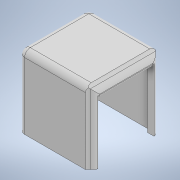
# Autodesk Inventor part: NEMA17_Shroud
Saved by Autodesk Inventor 2021 (Build 250183000, 183)
## iProperties
Created: 2021-10-06
Part Number: NEMA17_Shroud
Material: Generic
Document SubType Name: Modeling
Designer: Jorian Brusind
Density: 1 g/cm^3
Appearance: Default
Author: Jorian Brusind
Autodesk Inventor part; units mm, degrees
ref_plane "YZ Plane" through (0, 0, 0) normal (1, 0, 0) x (0, 1, 0)
ref_plane "XZ Plane" through (0, 0, 0) normal (0, 1, 0) x (-1, 0, 0)
ref_plane "XY Plane" through (0, 0, 0) normal (0, 0, 1) x (1, 0, 0)
sketch "Sketch1" plane through (0, 0, 0) normal (0, 1, 0) x (-1, 0, 0)
  line L0 (0, 0) -> (55, 0)
  line L1 (55, 0) -> (55, -55)
  line L2 (55, -55) -> (0, -55)
  line L3 (0, -58) -> (58, -58)
  line L4 (58, -58) -> (58, 3)
  line L5 (58, 3) -> (0, 3)
  line L6 (0, 3) -> (0, 0)
  line L7 (0, -55) -> (0, -58)
  dimension "d0" = 55
  dimension "d1" = 55
  dimension "d2" = 3
  constraints: 16 end point, 3 equal length, 2 perpendicular, 1 horizontal, 1 vertical, 2 other
  measures "d0" distance of L1.end L2.end
  measures "d1" distance of L0.end L1.end
  measures "d2" distance between parallel lines of L1 L4
extrude "Extrusion1" add sketch "Sketch1" along normal blind 60
sketch "Sketch2" plane through (0, 60, 0) normal (0, 1, 0) x (1, 0, 0)
  line L0 (-58, 58) -> (-58, -3) projected
  line L1 (0, 55) -> (0, 58) projected
  line L2 (-58, -3) -> (0, -3)
  line L3 (0, -3) -> (0, 58)
  line L4 (0, 58) -> (-58, 58)
  line L5 (-58, 58) -> (-58, -3)
  point P0 (0, 0)
  constraints: 8 end point, 2 parallel, 1 horizontal, 1 perpendicular
extrude "Extrusion2" add sketch "Sketch2" along normal blind 3
ref_plane "Work Plane1" through (0, -5, 0) normal (0, -1, 0) x (1, 0, 0)
ref_plane "Work Plane2" through (5, 60, 0) normal (1, 0, 0) x (0, 0, -1)
sketch "Sketch4" plane through (5, 60, 0) normal (1, 0, 0) x (0, 0, -1)
  line L0 (58, 3) -> (-3, 3) projected
  line L1 (27.5, 3) -> (27.5, -7)
  line L2 (0, -60) -> (0, 0) projected
  line L3 (0, -30) -> (3, -30)
  line L4 (55, -60) -> (55, 0) projected
  line L5 (55, -30) -> (52, -30)
  line L6 (52, -30) -> (52, -7)
  line L7 (52, -7) -> (27.5, -7)
  line L8 (27.5, -7) -> (3, -7)
  line L9 (3, -7) -> (3, -30)
  line L10 (3, -30) -> (3, -60)
  line L11 (0, -60) -> (55, -60) projected
  line L12 (52, -30) -> (52, -60)
  line L13 (52, -60) -> (55, -60)
  line L14 (3, -60) -> (0, -60)
  line L15 (0, -60) -> (0, -30)
  line L16 (0, 0) -> (55, 0) projected
  line L17 (0, -30) -> (0, 0)
  line L18 (0, 0) -> (55, 0)
  line L19 (55, 0) -> (55, -60)
  dimension "d26" = 10
  dimension "d27" = 3
  dimension "d28" = 3
  constraints: 30 end point, 5 point on line, 4 perpendicular, 3 collinear, 3 midpoint, 2 horizontal, 2 vertical
  measures "d26" distance of L1.start L1.end
  measures "d27" distance of L3.start L3.end
  measures "d28" distance of L5.start L5.end
extrude "Extrusion4" add sketch "Sketch4" against normal blind 6 contours L16 L4 L5 L6 L7 L1 | L1 L8 L9 L3 L2 L16 | L3 L10 L11 L2 | L4 L11 L12 L5
fillet "Fillet8" radius 6 3 edges at (0, 60, -27.5) (0, 30, -55) (0, 30, 0)
fillet "Fillet9" radius 6 3 edges at (5, 30.0016, 0.0032) (5, 60.0032, -27.5) (5, 30.0016, -55.0032)
fillet "Fillet10" radius 2 4 edges at (4.9656, 53, -51.3654) (4.9656, 53, -3.6346) (5, 53, -27.5) (-1, 53, -27.5)
fillet "Fillet11" radius 5 3 edges at (-29, 63, 3) (-29, 63, -58) (-58, 63, -27.5)
fillet "Fillet12" radius 5 4 edges at (-56.5355, 61.5355, 1.5355) (-58, 29, 3) (-56.5355, 61.5355, -56.5355) (-58, 29, -58)
body "Solid1"
